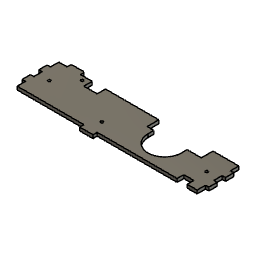
move_base_sidewall_2R (Autodesk Fusion 360 design; units mm, degrees)
Autodesk Fusion 360 part; units mm, degrees
note: some values were not read from the file. Set by a fixed rule: which sketch regions a step uses.
sketch "スケッチ1" plane through (0, 0, 0) normal (0, 1, 0) x (1, 0, 0)
  line L0 (-20, -14) -> (-20, -41)
  line L1 (-20, -41) -> (20, -41)
  line L2 (20, -41) -> (20, -14)
  line L3 (20, -14) -> (37, -14)
  line L4 (37, -14) -> (37, 0)
  line L5 (37, 0) -> (68, 0)
  line L6 (68, 0) -> (68, -10)
  line L7 (68, -10) -> (72, -10)
  line L8 (72, -10) -> (72, -20)
  line L9 (72, -20) -> (68, -20)
  line L10 (68, -20) -> (68, -30)
  line L11 (68, -30) -> (72, -30)
  line L12 (72, -30) -> (72, -40)
  line L13 (72, -40) -> (68, -40)
  line L14 (68, -40) -> (68, -50)
  line L15 (68, -50) -> (-148, -50)
  line L16 (-148, 0) -> (-28, 0)
  line L17 (-148, 0) -> (-148, -10)
  line L18 (-148, -10) -> (-152, -10)
  line L19 (-152, -10) -> (-152, -20)
  line L20 (-152, -20) -> (-148, -20)
  line L21 (-148, -20) -> (-148, -30)
  line L22 (-148, -30) -> (-152, -30)
  line L23 (-152, -30) -> (-152, -40)
  line L24 (-152, -40) -> (-148, -40)
  line L25 (-148, -40) -> (-148, -50)
  line L26 (-108, 0) -> (-92, 0)
  line L27 (-92, 0) -> (-92, -10)
  line L28 (-92, -10) -> (-108, -10)
  line L29 (-108, -10) -> (-108, 0)
  line L30 (-68, -50) -> (-52, -50)
  line L31 (-52, -50) -> (-52, -55)
  line L32 (-52, -55) -> (-68, -55)
  line L33 (-68, -55) -> (-68, -50)
  line L34 (-138, 0) -> (-122, 0)
  line L35 (-122, 0) -> (-122, 5)
  line L36 (-122, 5) -> (-138, 5)
  line L37 (-138, 5) -> (-138, 0)
  line L38 (56, -50) -> (44, -50)
  line L39 (44, -50) -> (44, -42)
  line L40 (44, -42) -> (56, -42)
  line L41 (56, -42) -> (56, -50)
  line L42 (-28, 0) -> (-28, -14)
  line L43 (-28, -14) -> (-20, -14)
  point P0 (-100, 0)
  point P1 (-130, 0)
  point P2 (-60, -50)
  dimension "d9" = 20
  dimension "d10" = 14
  dimension "d11" = 68
  dimension "d12" = 4
  dimension "d13" = 10
  dimension "d14" = 10
  dimension "d15" = 10
  dimension "d16" = 10
  dimension "d17" = 10
  dimension "d19" = 17
  dimension "d34" = 4
  dimension "d37" = 216
  dimension "d40" = 100
  dimension "d41" = 10
  dimension "d42" = 16
  dimension "d43" = 5
  dimension "d44" = 16
  dimension "d45" = 60
  dimension "d46" = 130
  dimension "d50" = 12
  dimension "d51" = 12
  dimension "d52" = 8
  dimension "d53" = 41
  dimension "d54" = 20
  dimension "d55" = 8
  constraint vertical L0
  constraint perpendicular L0 L1
  constraint perpendicular L1 L2
  constraint perpendicular L2 L3
  constraint perpendicular L1 L4
  constraint perpendicular L4 L5
  constraint perpendicular L5 L6
  constraint perpendicular L6 L7
  constraint perpendicular L7 L8
  constraint perpendicular L8 L9
  constraint perpendicular L9 L10
  constraint perpendicular L8 L11
  constraint perpendicular L9 L12
  constraint perpendicular L12 L13
  constraint perpendicular L13 L14
  constraint perpendicular L14 L15
  constraint perpendicular L0 L16
  constraint collinear L6 L10
  constraint collinear L10 L14
  constraint collinear L8 L12
  constraint horizontal origin L4.end
  constraint horizontal origin L16.end
  constraint perpendicular L16 L17
  constraint perpendicular L17 L18
  constraint perpendicular L16 L19
  constraint perpendicular L19 L20
  constraint perpendicular L20 L21
  constraint perpendicular L21 L22
  constraint perpendicular L22 L23
  constraint perpendicular L23 L24
  constraint perpendicular L15 L25
  constraint collinear L17 L21
  constraint collinear L21 L25
  constraint collinear L19 L23
  constraint collinear L7 L18
  constraint collinear L9 L20
  constraint collinear L11 L22
  constraint collinear L13 L24
  constraint horizontal L26
  constraint vertical L27
  constraint horizontal L28
  constraint vertical L29
  constraint midpoint L26 P0
  constraint coincident L16 P0
  constraint horizontal L30
  constraint vertical L31
  constraint horizontal L32
  constraint vertical L33
  constraint horizontal L34
  constraint vertical L35
  constraint horizontal L36
  constraint vertical L37
  constraint midpoint L34 P1
  constraint midpoint L30 P2
  constraint coincident L15 P2
  constraint coincident L16 P1
  constraint equal L33 L35
  constraint equal L32 L36
  constraint horizontal L38
  constraint vertical L39
  constraint horizontal L40
  constraint vertical L41
  constraint coincident L15 L38.start
  constraint perpendicular L16 L42
  constraint perpendicular L0 L43
  constraint coincident L0.start L43.end
  constraint collinear L3 L43
  measures "d9" distance of origin L2
  measures "d10" distance of L3.end L4.end
  measures "d11" distance of origin L6
  measures "d12" distance of L6.end L7.end
  measures "d13" distance of L5.end L6.end
  measures "d14" distance of L7.end L8.end
  measures "d15" distance of L9.end L10.end
  measures "d16" distance of L11.end L12.end
  measures "d17" distance of L13.end L14.end
  measures "d19" distance of L2.end L3.end
  measures "d34" distance of L17.end L18.end
  measures "d37" distance of L6 L17
  measures "d40" distance of origin P0
  measures "d41" distance of L26.start L28.end
  measures "d42" distance of L27.end L28.end
  measures "d43" distance of L30.start L32.end
  measures "d44" distance of L31.end L32.end
  measures "d45" horizontal distance of origin P2
  measures "d46" distance of origin P1
  measures "d50" distance of L39.end L40.end
  measures "d51" distance of L14 L41
  measures "d52" distance of L38.end L39.end
  measures "d53" distance of L1 L16
  measures "d54" distance of origin L0
  measures "d55" distance of L0 L42
extrude "押し出し1" add sketch "スケッチ1" along normal blind 4 contours L0 L1 L2 L3 L4 L5 L6 L7 L8 L9 L10 L11 L12 L13 L14 L15 L16 L17 L18 L19 L20 L21 L22 L23 L24 L25 L27 L28 L29 L30 L34 L39 L40 L41 L42 L43 | L16 L34 L35 L36 L37 | L15 L30 L31 L32 L33
sketch "スケッチ2" plane through (0, 4, 0) normal (0, 1, 0) x (-1, 0, 0)
  line L0 (-56, 50) -> (-68, 50)
  line L1 (-68, 50) -> (-68, 40)
  line L2 (-68, 40) -> (-72, 40)
  line L3 (-72, 40) -> (-72, 30)
  line L4 (-72, 30) -> (-68, 30)
  line L5 (-68, 30) -> (-68, 20)
  line L6 (-68, 20) -> (-72, 20)
  line L7 (-72, 20) -> (-72, 10)
  line L8 (-72, 10) -> (-68, 10)
  line L9 (-68, 10) -> (-68, 0)
  line L10 (-68, 0) -> (-37, 0)
  line L11 (-37, 0) -> (-37, 14)
  line L12 (-37, 14) -> (-20, 14)
  line L13 (-20, 14) -> (-20, 41)
  line L14 (-20, 41) -> (20, 41)
  line L15 (20, 41) -> (20, 14)
  line L16 (138, 0) -> (148, 0)
  line L17 (-54.5, 25) -> (-68, 25)
  line L18 (60, 36.5) -> (115, 5)
  line L19 (148, 0) -> (148, 10)
  line L20 (148, 10) -> (152, 10)
  line L21 (152, 10) -> (152, 20)
  line L22 (152, 20) -> (148, 20)
  line L23 (148, 20) -> (148, 30)
  line L24 (148, 30) -> (152, 30)
  line L25 (152, 30) -> (152, 40)
  line L26 (152, 40) -> (148, 40)
  line L27 (148, 40) -> (148, 50)
  line L28 (148, 25) -> (134.5, 25)
  line L29 (92, 0) -> (92, 10)
  line L30 (92, 10) -> (108, 10)
  line L31 (108, 10) -> (108, 0)
  line L32 (122, 0) -> (122, -5)
  line L33 (122, -5) -> (138, -5)
  line L34 (138, -5) -> (138, 0)
  line L35 (68, 50) -> (68, 55)
  line L36 (68, 55) -> (52, 55)
  line L37 (52, 55) -> (52, 50)
  line L38 (52, 50) -> (-44, 50)
  line L39 (108, 0) -> (122, 0)
  line L40 (-44, 50) -> (-44, 42)
  line L41 (-44, 42) -> (-56, 42)
  line L42 (-56, 42) -> (-56, 50)
  line L43 (148, 50) -> (68, 50)
  line L44 (20, 14) -> (28, 14)
  line L45 (28, 14) -> (28, 0)
  line L46 (28, 0) -> (92, 0)
  dimension "d24" = 13.5
  dimension "d25" = 5
  dimension "d27" = 13.5
  dimension "d38" = 60
  dimension "d39" = 115
  constraint midpoint L5 L17.end
  constraint perpendicular L5 L17
  constraint horizontal L28
  constraint midpoint L23 L28.start
  constraint equal L17 L28
  measures "d24" distance of L17.start L17.end
  measures "d25" vertical distance of origin L18.end
  measures "d27" distance of L0 L18.start
  measures "d34" distance of origin
  measures "d38" horizontal distance of origin L18.start
  measures "d39" horizontal distance of origin L18.end
hole "穴1" at (-115, 4, 5) at (-60, 4, 36.5) at (54.5, 4, 25) at (-134.5, 4, 25) direction (0, -1, 0) diameter 3.2 end through all
fillet "フィレット1" radius 20 2 edges at (20, 2, 41) (-20, 2, 41)
chamfer "面取り1" distance 1 angle 45 2 edges at (-138, 2, -5) (-122, 2, -5)
